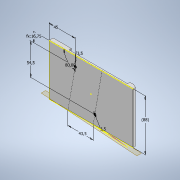
# Autodesk Inventor part: PedalHolder
Saved by Autodesk Inventor 2021 (Build 250183000, 183)
## iProperties
Created: 2021-02-09
Part Number: PedalHolder
Material: Generic
Document SubType Name: Modeling
Designer: Viktor
Density: 1 g/cm^3
Appearance: Default
Author: Viktor
## iProperties of the stored document _3DPrint.ipt
Created: 2021-02-09
Part Number: _3DPrint
Material: Generic
Document SubType Name: Modeling
Designer: Viktor
Density: 1 g/cm^3
Appearance: Default
Author: Viktor
Autodesk Inventor part; units mm, degrees
ref_plane "YZ Plane" through (0, 0, 0) normal (1, 0, 0) x (0, 1, 0)
ref_plane "XZ Plane" through (0, 0, 0) normal (0, 1, 0) x (-1, 0, 0)
ref_plane "XY Plane" through (0, 0, 0) normal (0, 0, 1) x (1, 0, 0)
sketch "Sketch1" plane through (0, 0, 0) normal (0, 0, 1) x (1, 0, 0)
  line L0 (-72.5, -44) -> (72.5, -44)
  line L1 (72.5, -44) -> (72.5, 44)
  line L2 (72.5, 44) -> (-72.5, 44)
  line L3 (-72.5, 44) -> (-72.5, -44)
  line L4 (-72.5, -44) -> (72.5, 44) construction
  line L5 (72.5, -44) -> (-72.5, 44) construction
  point P0 (0, 0)
  dimension "d0" = 145
  dimension "d1" = 88
  constraints: 12 end point, 2 midpoint, 2 parallel, 1 horizontal, 1 perpendicular
  measures "d0" distance of L1.end L2.end
  measures "d1" distance between parallel lines of L0 L2
extrude "Extrusion1" add sketch "Sketch1" along normal blind 7
sketch "Sketch2" plane through (0, 0, 7) normal (0, 0, 1) x (1, 0, 0)
  line L0 (-24.5465, 44) -> (-40.0633, -44) construction
  line L1 (18.9535, 44) -> (3.4367, -44) construction
  line L2 (72.5, 44) -> (-72.5, 44) projected
  line L3 (-72.5, -44) -> (72.5, -44) projected
  circle A0 centre (6.3902, -27.25) radius 1.75
  circle A1 centre (-27.5, 27.25) radius 1.75
  line L4 (-72.5, 44) -> (-72.5, -44) projected
  point P0 (0, 0)
  dimension "d4" = 80
  dimension "d5" = 43.5
  dimension "d6" = 3.5
  dimension "d7" = 3.5
  dimension "d8" = 54.5
  dimension "d9" = 16.75
  dimension "d10" = 88
  dimension "d11" = 45
  constraints: 6 point on line, 4 end point, 2 centre point, 1 parallel
  measures "d4" angle of L2 L0
  measures "d5" distance of L1.end L0.end
  measures "d6" diameter of A1
  measures "d7" diameter of A0
  measures "d8" vertical distance of A0.centre A1.centre
  measures "d9" distance from line of L2 A1.centre
  measures "d10" distance between parallel lines of L2 L3
  measures "d11" distance from line of L4 A1.centre
sketch "Sketch3" plane through (0, 0, 0) normal (0, 0, -1) x (-1, 0, 0)
  line L0 (72.5, -44) -> (-72.5, -44) projected
  line L1 (-72.5, 44) -> (72.5, 44) projected
  line L2 (40, -44) -> (-60, -44)
  line L3 (-60, -44) -> (-60, 44)
  line L4 (-60, 44) -> (40, 44)
  line L5 (40, 44) -> (40, -44)
  line L6 (-72.5, -44) -> (-72.5, 44) projected
  line L7 (72.5, 44) -> (72.5, -44) projected
  point P0 (0, 0)
  point P1 (40, 44)
  point P2 (-60, -44)
  dimension "d14" = 100
  dimension "d15" = 145
  dimension "d16" = 32.5
  constraints: 8 end point, 2 parallel, 2 point on line, 1 horizontal, 1 perpendicular
  measures "d14" distance between parallel lines of L3 L5
  measures "d15" distance between parallel lines of L6 L7
  measures "d16" distance between parallel lines of L5 L7
extrude "Extrusion3" cut sketch "Sketch3" against normal blind 4 contours L0 L3 L1 L5
sketch "Sketch5" plane through (-72.5, -44, 7) normal (0, -1, 0) x (1, 0, 0)
  line L0 (145, -7) -> (132.5, -7) projected
  arc A0 (139, -7) -> (145, -4) centre (128.6677, 21.1646) ccw
  line L1 (145, -7) -> (145, 0) projected
  line L2 (132.5, -7) -> (145, -7) projected
  line L3 (132.5, -3) -> (132.5, -7) projected
  point P0 (72.5, -7)
  point P1 (132.5, -4)
  point P2 (139, -7)
  dimension "d25" = 4
  dimension "d26" = 6.5
  dimension "d27" = 30
  constraints: 2 point on circle, 2 point on line, 1 centre point
  measures "d25" distance of L1.end A0.end
  measures "d26" distance from line of L3 A0.start
  measures "d27" radius of A0
extrude "Extrusion5" cut sketch "Sketch5" against normal through all
chamfer "Chamfer1" distance 0.5 angle 45 4 edges at (-72.5, 0, 7) (0, 44, 7) (72.5, 0, 7) (0, -44, 7)
sketch "Sketch7" plane through (0, 0, 4) normal (0, 0, -1) x (-1, 0, 0)
  line L0 (72.5, -44) -> (40, -44) projected
  line L1 (40, 44) -> (72.5, 44) projected
  line L2 (40, -44) -> (-60, -44) projected
  line L3 (40, -44) -> (40, 44)
  line L4 (40, -44) -> (47, -44)
  line L5 (47, -44) -> (41, 44)
  line L6 (41, 44) -> (40, 44)
  point P0 (0, 0)
  dimension "d34" = 7
  dimension "d35" = 1
  constraints: 8 end point, 2 point on line, 1 collinear, 1 perpendicular
  measures "d34" distance from line of L3 L4.end
  measures "d35" distance from line of L3 L5.end
extrude "Extrusion6" cut sketch "Sketch7" along normal through all
sketch "Sketch8" plane through (60, -44, 0) normal (0, -1, 0) x (1, 0, 0)
  point P0 (-60, 0)
ref_plane "Work Plane1" through (-47, -44, 2) normal (0.068, 0.9977, 0) x (0, 0, 1)
sketch "Sketch9" plane through (-47, -44, 2) normal (0.068, 0.9977, 0) x (0, 0, 1)
  line L0 (2, 0) -> (2, 106.7522) projected
  line L1 (2, 0) -> (-1, 20) construction
  line L2 (-1, 20) -> (-1, 54) construction
  line L3 (2, 106.7522) -> (2, 100.7661) projected
  line L4 (-1, 54) -> (2, 106.7522) construction
  spline S0 degree 3 poles (2, 0) (-1, 20) (-1, 54) (2, 106.7522) knots 1 1 1 1 2 2 2 2
  point P0 (-2, 43.8981)
  constraints: 1 vertical, 3 other
equation "\"d9\" = -0.5 * d8 + 0.5 * d10"
body "Solid1"
